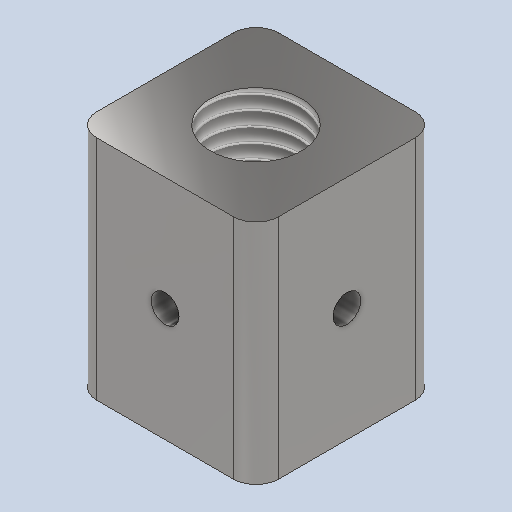
# Autodesk Inventor part: leadscrew
Saved by Autodesk Inventor 2025.4 (Build 294407000, 407)
## iProperties
Created: 2026-03-22
Part Number: leadscrew
Material: Steel, Cast
Document SubType Name: Modeling
Designer: hp
Density: 7.85 g/cm^3
Appearance: Semi-Polished
Author: hp
Autodesk Inventor part; units mm, degrees
ref_plane "YZ Plane" through (0, 0, 0) normal (1, 0, 0) x (0, 1, 0)
ref_plane "XZ Plane" through (0, 0, 0) normal (0, 1, 0) x (-1, 0, 0)
ref_plane "XY Plane" through (0, 0, 0) normal (0, 0, 1) x (1, 0, 0)
sketch "Sketch1" plane through (0, 0, 0) normal (0, 1, 0) x (-1, 0, 0)
  circle A0 centre (0, 0) radius 4
  line L0 (6, 8) -> (-6, 8)
  line L1 (-8, 6) -> (-8, -6)
  line L2 (-6, -8) -> (6, -8)
  line L3 (8, -6) -> (8, 6)
  line L4 (8, 8) -> (-8, -8) construction
  line L5 (-8, 8) -> (8, -8) construction
  arc A1 (8, 6) -> (6, 8) centre (6, 6) ccw
  arc A2 (6, -8) -> (8, -6) centre (6, -6) ccw
  arc A3 (-8, -6) -> (-6, -8) centre (-6, -6) ccw
  arc A4 (-6, 8) -> (-8, 6) centre (-6, 6) ccw
  dimension "d0" = 8
  dimension "d1" = 16
  dimension "d2" = 16
  dimension "d5" = 2
  constraints: 12 end point, 8 point on circle, 8 point on line, 8 tangent, 5 centre point, 3 equal radius, 2 midpoint, 2 parallel, 1 coincident, 1 horizontal, 1 perpendicular
  measures "d0" diameter of A0
  measures "d1" distance of L5.end L4.end
  measures "d2" distance of L4.end L5.start
  measures "d5" radius of A1
extrude "Extrusion1" add sketch "Sketch1" along normal blind 20
sketch "Sketch2" plane through (-6, 0, 8) normal (0, 0, 1) x (1, 0, 0)
  line L0 (0, 0) -> (12, 0) projected
  line L1 (12, 0) -> (12, 20) projected
  line L2 (0, 20) -> (12, 20) projected
  line L3 (0, 0) -> (0, 20) projected
  point P0 (6, 0)
  point P1 (6, 10)
  dimension "d6" = 6
  measures "d6" distance from line of point (6, 10) L3
hole "Hole1" at (0, 10, 8) direction (0, 0, -1) diameter 2.45 depth 3 tip angle 118
pattern_circular "Circular Pattern1" count 4 over 360 about axis through (0, -10, 0) along (0, 1, 0) of "Hole1"
thread "Thread1" size "M8x1.25" class "6H" standard "ANSI Metric M Profile" full length
body "Solid1"
